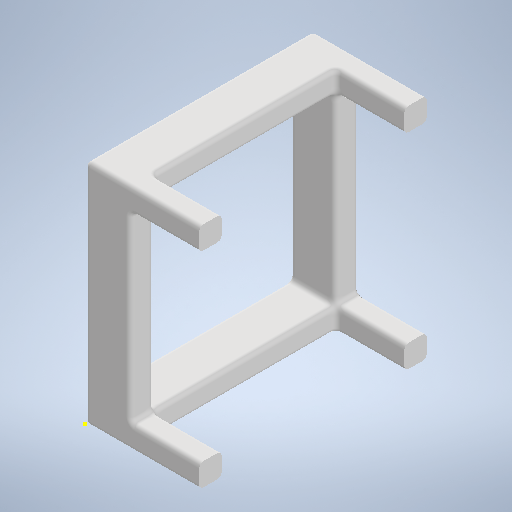
# Autodesk Inventor part: Pièce1
Saved by Autodesk Inventor 2025.2 (Build 292293000, 293)
## iProperties
Created: 2025-02-15
Part Number: Pièce1
Material: Générique
Document SubType Name: Modeling
Designer: antoi
Density: 1 g/cm^3
Appearance: Par défaut
Author: antoi
Autodesk Inventor part; units mm, degrees
ref_plane "YZ Plane" through (0, 0, 0) normal (1, 0, 0) x (0, 1, 0)
ref_plane "XZ Plane" through (0, 0, 0) normal (0, 1, 0) x (-1, 0, 0)
ref_plane "XY Plane" through (0, 0, 0) normal (0, 0, 1) x (1, 0, 0)
sketch "Esquisse1" plane through (0, 0, 0) normal (1, 0, 0) x (0, 1, 0)
  line L0 (0, 0) -> (100, 0)
  line L1 (100, 0) -> (100, -100)
  line L2 (100, -100) -> (0, -100)
  line L3 (0, -100) -> (0, 0)
  dimension "d0" = 100
  dimension "d1" = 100
  constraints: 8 end point, 2 parallel, 1 horizontal, 1 perpendicular
  measures "d0" distance of L1.end L2.end
  measures "d1" distance of L0.end L1.end
extrude "Extrusion1" add sketch "Esquisse1" against normal blind 20
sketch "Esquisse2" plane through (0, 0, 0) normal (1, 0, 0) x (0, 0, -1)
  line L0 (10, 10) -> (90, 10)
  line L1 (90, 10) -> (90, 90)
  line L2 (90, 90) -> (10, 90)
  line L3 (10, 90) -> (10, 10)
  point P0 (0, 0)
  dimension "d4" = 80
  dimension "d5" = 80
  constraints: 8 end point, 2 parallel, 1 horizontal, 1 perpendicular
  measures "d4" distance of L2.end L1.end
  measures "d5" distance of L1.end L0.end
extrude "Extrusion2" cut sketch "Esquisse2" against normal up to surface (20 mm away)
sketch "Esquisse3" plane through (0, 0, 0) normal (1, 0, 0) x (0, 0, -1)
  line L0 (10, 10) -> (10, 90) projected
  line L1 (0, 0) -> (10, 0)
  line L2 (10, 0) -> (10, 10)
  line L3 (10, 10) -> (0, 10)
  line L4 (0, 10) -> (0, 0)
  constraints: 8 end point, 2 parallel, 1 horizontal, 1 perpendicular
extrude "Extrusion3" add sketch "Esquisse3" along normal blind 30
sketch "Esquisse5" plane through (-20, 0, 0) normal (-1, 0, 0) x (0, 0, 1)
  circle A0 centre (-5, 5) radius 1.6952
  point P0 (0, 0)
  constraints: 1 centre point
hole "Perçage1" at (-20, 5, -5) direction (1, 0, 0) diameter 5.9175 depth 5 thread size "M7x1" class "6H" standard "ISO Metric profile"
pattern_linear "Réseau rectangulaire4" count 2 spacing 90 along (0, 1, 0) count 2 spacing 90 along (0, 0, -1) of "Perçage1", "Extrusion3"
fillet "Congé4" radius 2 44 edges at (-20, 50, -100) (-20, 50, -90) (-20, 90, -50) (-20, 100, -50) (-20, 50, -10) (-20, 50, 0) (-20, 10, -50) (-20, 0, -50) (0, 0, -50) (0, 10, -50) (0, 50, -100) (0, 50, -90) (0, 90, -50) (0, 100, -50) (0, 50, -10) (0, 50, 0) (15, 0, -10) (15, 10, -10) (5, 0, 0) (15, 10, 0) (15, 0, -90) (5, 0, -100) (15, 10, -100) (15, 10, -90) (15, 90, -100) (15, 90, -90) (15, 100, -90) (5, 100, -100) (15, 100, -10) (15, 90, -10) (15, 90, 0) (0, 95, -10) (5, 100, 0) (0, 90, -5) (0, 90, -95) (0, 95, -90) (0, 10, -95) (0, 5, -90) (0, 5, -10) (0, 10, -5) (-10, 10, -10) (-10, 10, -90) (-10, 90, -90) (-10, 90, -10)
